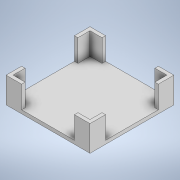
# Autodesk Inventor part: servoBracket
Saved by Autodesk Inventor 2020 (Build 240168000, 168)
## iProperties
Created: 2020-04-05
Part Number: servoBracket
Material: Generic
Document SubType Name: Modeling
Designer: jared.jones280
Density: 1 g/cm^3
Appearance: Default
Author: jared.jones280
Autodesk Inventor part; units mm, degrees
ref_plane "YZ Plane" through (0, 0, 0) normal (1, 0, 0) x (0, 1, 0)
ref_plane "XZ Plane" through (0, 0, 0) normal (0, 1, 0) x (-1, 0, 0)
ref_plane "XY Plane" through (0, 0, 0) normal (0, 0, 1) x (1, 0, 0)
sketch "Sketch1" plane through (0, 0, 0) normal (0, 1, 0) x (-1, 0, 0)
  line L0 (0, 0) -> (-44, 0)
  line L1 (-44, 0) -> (-44, -44)
  line L2 (-44, -44) -> (0, -44)
  line L3 (0, -44) -> (0, 0)
  line L4 (2, 2) -> (-46, 2)
  line L5 (-46, 2) -> (-46, -46)
  line L6 (-46, -46) -> (2, -46)
  line L7 (2, -46) -> (2, 2)
  dimension "d0" = 44
  dimension "d1" = 44
  dimension "d2" = 48
  dimension "d3" = 48
  dimension "d4" = 2
  dimension "d5" = 2
  constraints: 16 end point, 4 parallel, 2 horizontal, 2 perpendicular
  measures "d0" distance of L2.end L1.end
  measures "d1" distance of L1.end L0.end
  measures "d2" distance of L6.end L5.end
  measures "d3" distance of L5.end L4.end
  measures "d4" distance between parallel lines of L7 L3
  measures "d5" distance between parallel lines of L2 L6
extrude "Extrusion1" add sketch "Sketch1" along normal blind 12.7
sketch "Sketch2" plane through (0, 0, 0) normal (0, -1, 0) x (1, 0, 0)
  line L0 (46, 2) -> (46, -46) projected
  line L1 (-2, 2) -> (46, 2) projected
  line L2 (-2, -46) -> (-2, 2) projected
  line L3 (46, -46) -> (-2, -46) projected
  point P0 (0, 0)
extrude "Extrusion2" add sketch "Sketch2" along normal blind 2
sketch "Sketch3" plane through (0, 0, 0) normal (0, 1, 0) x (1, 0, 0)
  line L0 (-2, -2) -> (46, -2) projected
  line L1 (-2, 46) -> (-2, -2) projected
  line L2 (46, 46) -> (-2, 46) projected
  line L3 (46, -2) -> (46, 46) projected
  line L4 (37.11, -2) -> (6.89, -2)
  line L5 (6.89, -2) -> (6.89, 46)
  line L6 (6.89, 46) -> (37.11, 46)
  line L7 (37.11, 46) -> (37.11, -2)
  line L8 (-2, -2) -> (-2, 46) projected
  line L9 (-2, 6.89) -> (46, 6.89)
  line L10 (46, 6.89) -> (46, 37.11)
  line L11 (46, 37.11) -> (-2, 37.11)
  line L12 (-2, 37.11) -> (-2, 6.89)
  point P0 (0, 0)
  point P1 (37.11, 37.11)
  point P2 (37.11, 6.89)
  point P3 (6.89, 6.89)
  point P4 (6.89, 37.11)
  point P5 (-2, 37.11)
  dimension "d10" = 8.89
  dimension "d11" = 8.89
  dimension "d12" = 8.89
  dimension "d13" = 8.89
  constraints: 16 end point, 4 parallel, 4 point on line, 2 horizontal, 2 perpendicular
  measures "d10" distance between parallel lines of L1 L5
  measures "d11" distance between parallel lines of L0 L9
  measures "d12" distance between parallel lines of L3 L7
  measures "d13" distance between parallel lines of L11 L2
extrude "Extrusion3" cut sketch "Sketch3" along normal blind 2 contours L5 L9 L7 L0 | L1 L11 L5 L9 | L7 L11 L3 L9 | L5 L2 L7 L11
extrude "Extrusion4" cut sketch "Sketch3" along normal blind 76.2 contours L5 L9 L7 L0 | L1 L11 L5 L9 | L7 L11 L3 L9 | L5 L2 L7 L11
body "Solid1"
